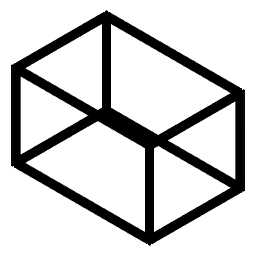
PONG_Frame v2 (Autodesk Fusion 360 design; units mm, degrees)
Autodesk Fusion 360 part; units mm, degrees
sketch "スケッチ1" plane through (0, 0, 0) normal (0, 1, 0) x (1, 0, 0) in component "MisumiFrame20x20 v1"
  line L0 (2.1, 0) -> (4, 0)
  line L1 (10, 3) -> (10, 9)
  line L2 (9, 10) -> (3, 10)
  line L3 (0, 4) -> (0, 2.1)
  arc A0 (10, 9) -> (9, 10) centre (9, 9) ccw
  line L4 (10, 3) -> (8, 3)
  line L5 (8, 3) -> (8, 6)
  line L6 (8, 6) -> (4, 2)
  line L7 (4, 2) -> (4, 0)
  line L8 (3, 10) -> (3, 8)
  line L9 (3, 8) -> (6, 8)
  line L10 (6, 8) -> (2, 4)
  line L11 (2, 4) -> (0, 4)
  arc A1 (2.1, 0) -> (0, 2.1) centre (0, 0) ccw
  dimension "d3" = 1
  dimension "d4" = 4.2
  constraint horizontal L0
  constraint vertical L1
  constraint horizontal L2
  constraint vertical L3
  constraint tangent L2 A0
  constraint tangent L1 A0
  constraint perpendicular L1 L4
  constraint perpendicular L4 L5
  constraint perpendicular L0 L7
  constraint perpendicular L2 L8
  constraint perpendicular L8 L9
  constraint perpendicular L3 L11
  constraint coincident A1.centre origin
  measures "d3" radius of A0
  measures "d4" diameter of A1
extrude "押し出し1" add sketch "スケッチ1" along normal blind 400 makes body 1 in component "MisumiFrame20x20 v1"
mirror "ミラー1" about plane through (2.1, 0, 0) normal (0, 0, -1) of bodies 1 makes body 2 in component "MisumiFrame20x20 v1"
mirror "ミラー2" about plane through (0, 0, -4) normal (1, 0, 0) of bodies 1 2 makes body 3 at (-7, 133.3333, -10) makes body 4 at (-7, 133.3333, 10) in component "MisumiFrame20x20 v1"
combine "結合1" operation add target body 4 tool bodies 3 1 2 in component "MisumiFrame20x20 v1"
copy_body "ボディのコピーと貼り付け1" bodies 4 makes body 5
sketch "スケッチ1 (2)" plane through (0, 0, 0) normal (0, 1, 0) x (1, 0, 0) in component "MisumiFrame20x20 v1 (1)"
  line L0 (2.1, 0) -> (4, 0)
  line L1 (10, 3) -> (10, 9)
  line L2 (9, 10) -> (3, 10)
  line L3 (0, 4) -> (0, 2.1)
  arc A0 (10, 9) -> (9, 10) centre (9, 9) ccw
  line L4 (10, 3) -> (8, 3)
  line L5 (8, 3) -> (8, 6)
  line L6 (8, 6) -> (4, 2)
  line L7 (4, 2) -> (4, 0)
  line L8 (3, 10) -> (3, 8)
  line L9 (3, 8) -> (6, 8)
  line L10 (6, 8) -> (2, 4)
  line L11 (2, 4) -> (0, 4)
  arc A1 (2.1, 0) -> (0, 2.1) centre (0, 0) ccw
  dimension "d3_1" = 1
  dimension "d4_1" = 4.2
  constraint horizontal L0
  constraint vertical L1
  constraint horizontal L2
  constraint vertical L3
  constraint tangent L2 A0
  constraint tangent L1 A0
  constraint perpendicular L1 L4
  constraint perpendicular L4 L5
  constraint perpendicular L0 L7
  constraint perpendicular L2 L8
  constraint perpendicular L8 L9
  constraint perpendicular L3 L11
  constraint coincident A1.centre origin
  measures "d3_1" radius of A0
  measures "d4_1" diameter of A1
extrude "押し出し1'" add sketch "スケッチ1 (2)" along normal blind 600 separate body makes body 6 in component "MisumiFrame20x20 v1 (1)"
mirror "ミラー1'" about plane through (2.1, 0, 0) normal (0, 0, -1) of bodies 6 makes body 7 in component "MisumiFrame20x20 v1 (1)"
mirror "ミラー2'" about plane through (0, 0, -4) normal (1, 0, 0) of bodies 6 7 makes body 8 at (-7, 400, -10) makes body 9 at (-7, 400, 10) in component "MisumiFrame20x20 v1 (1)"
combine "結合1'" operation add target body 9 tool bodies 6 8 7 in component "MisumiFrame20x20 v1 (1)"
move_body "位置合わせ1" bodies 9 to x (1, 0, 0) y (0, 1, 0) z (0, 0, 1) at (5.4474, -15.4474, 0) in component "MisumiFrame20x20 v1 (1)"
sketch "スケッチ1 (3)" plane through (0, 0, 0) normal (0, 1, 0) x (1, 0, 0) in component "MisumiFrame20x20 v1 (2)"
  line L0 (2.1, 0) -> (4, 0)
  line L1 (10, 3) -> (10, 9)
  line L2 (9, 10) -> (3, 10)
  line L3 (0, 4) -> (0, 2.1)
  arc A0 (10, 9) -> (9, 10) centre (9, 9) ccw
  line L4 (10, 3) -> (8, 3)
  line L5 (8, 3) -> (8, 6)
  line L6 (8, 6) -> (4, 2)
  line L7 (4, 2) -> (4, 0)
  line L8 (3, 10) -> (3, 8)
  line L9 (3, 8) -> (6, 8)
  line L10 (6, 8) -> (2, 4)
  line L11 (2, 4) -> (0, 4)
  arc A1 (2.1, 0) -> (0, 2.1) centre (0, 0) ccw
  dimension "d3_2" = 1
  dimension "d4_2" = 4.2
  constraint horizontal L0
  constraint vertical L1
  constraint horizontal L2
  constraint vertical L3
  constraint tangent L2 A0
  constraint tangent L1 A0
  constraint perpendicular L1 L4
  constraint perpendicular L4 L5
  constraint perpendicular L0 L7
  constraint perpendicular L2 L8
  constraint perpendicular L8 L9
  constraint perpendicular L3 L11
  constraint coincident A1.centre origin
  measures "d3_2" radius of A0
  measures "d4_2" diameter of A1
extrude "押し出し1''" add sketch "スケッチ1 (3)" along normal blind 400 separate body makes body 10 in component "MisumiFrame20x20 v1 (2)"
mirror "ミラー1''" about plane through (2.1, 0, 0) normal (0, 0, -1) of bodies 10 makes body 11 in component "MisumiFrame20x20 v1 (2)"
mirror "ミラー2''" about plane through (0, 0, -4) normal (1, 0, 0) of bodies 10 11 makes body 12 at (-7, 133.3333, -10) makes body 13 at (-7, 133.3333, 10) in component "MisumiFrame20x20 v1 (2)"
combine "結合1''" operation add target body 13 tool bodies 11 12 10 in component "MisumiFrame20x20 v1 (2)"
move_body "位置合わせ1'" bodies 13 to x (1, 0, 0) y (0, 1, 0) z (0, 0, 1) at (0, -25.4474, -5.4474) in component "MisumiFrame20x20 v1 (2)"
copy_body "ボディのコピーと貼り付け2" bodies 5 makes body 14
move_body "移動1" bodies 14 to x (1, 0, 0) y (0, 1, 0) z (0, 0, 1) at (800, 0, 0)
move_body "位置合わせ1''" bodies 14 to x (1, 0, 0) y (0, 1, 0) z (0, 0, 1) at (-180, 0, 0)
copy_body "ボディのコピーと貼り付け3" bodies 13 body 13 seen with x (1, 0, 0) y (0, 0, -1) z (0, 1, 0) at (0, 15.4474, -35.4474) makes body 15
move_body "移動2" bodies 15 to x (1, 0, 0) y (0, 1, 0) z (0, 0, 1) at (860, 0, 0)
move_body "位置合わせ2" bodies 15 to x (1, 0, 0) y (0, 1, 0) z (0, 0, 1) at (-240, 0, 0)
copy_body "ボディのコピーと貼り付け4" bodies 9 body 9 seen with x (0, -1, 0) y (1, 0, 0) z (0, 0, 1) at (25.4474, 15.4474, 0) makes body 16
move_body "移動3" bodies 16 to x (1, 0, 0) y (0, 1, 0) z (0, 0, 1) at (0, 0, -450)
move_body "移動4" bodies 16 to x (1, 0, 0) y (0, 1, 0) z (0, 0, 1) at (0, 0, -175)
copy_body "ボディのコピーと貼り付け5" bodies 5 makes body 17
move_body "移動5" bodies 17 to x (1, 0, 0) y (0, 1, 0) z (0, 0, 1) at (0, 0, -600)
copy_body "ボディのコピーと貼り付け6" bodies 17 makes body 18
move_body "移動6" bodies 18 to x (1, 0, 0) y (0, 1, 0) z (0, 0, 1) at (850, 0, 0)
move_body "位置合わせ3" bodies 18 to x (1, 0, 0) y (0, 1, 0) z (0, 0, 1) at (-230, 0, 180)
move_body "位置合わせ4" bodies 16 to x (1, 0, 0) y (0, 1, 0) z (0, 0, 1) at (0, 0, 205)
move_body "位置合わせ5" bodies 17 to x (1, 0, 0) y (0, 1, 0) z (0, 0, 1) at (0, 0, 180)
copy_body "ボディのコピーと貼り付け7" bodies 15 16 13 9 body 13 seen with x (1, 0, 0) y (0, 0, -1) z (0, 1, 0) at (0, 15.4474, -35.4474) body 9 seen with x (0, -1, 0) y (1, 0, 0) z (0, 0, 1) at (25.4474, 15.4474, 0) makes body 19 makes body 20 makes body 21 makes body 22
move_body "移動7" bodies 19 20 21 22 to x (1, 0, 0) y (0, 1, 0) z (0, 0, 1) at (0, 300, 0)
move_body "位置合わせ6" bodies 20 to x (1, 0, 0) y (0, 1, 0) z (0, 0, 1) at (0, 80, 0)
move_body "位置合わせ7" bodies 21 to x (1, 0, 0) y (0, 1, 0) z (0, 0, 1) at (0, 80, 0)
move_body "位置合わせ8" bodies 19 to x (1, 0, 0) y (0, 1, 0) z (0, 0, 1) at (0, 80, 0)
move_body "位置合わせ9" bodies 22 to x (1, 0, 0) y (0, 1, 0) z (0, 0, 1) at (0, 80, 0)
component "MisumiFrame20x20 v1" placed x (1, 0, 0) y (0, 1, 0) z (0, 0, 1) at (0, 0, 0)
component "MisumiFrame20x20 v1 (1)" placed x (0, -1, 0) y (1, 0, 0) z (0, 0, 1) at (25.4474, 15.4474, 0)
component "MisumiFrame20x20 v1 (2)" placed x (1, 0, 0) y (0, 0, -1) z (0, 1, 0) at (0, 15.4474, -35.4474)
equation "d5 = 長さ"
equation "高さ = 400 mm" comment "フレーム長"
equation "d5_1 = 長さ"
equation "奥行 = 600 mm" comment "フレーム長"
equation "d5_2 = 長さ"
equation "幅 = 400 mm" comment "フレーム長"
